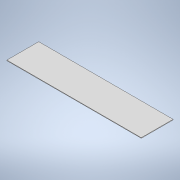
# Autodesk Inventor part: placa grande
Saved by Autodesk Inventor 2021.2 (Build 252289000, 289)
## iProperties
Created: 2021-04-23
Part Number: placa grande
Material: Genérico
Document SubType Name: Modeling
Designer: equip
Density: 1 g/cm^3
Appearance: Valor por defecto
Author: equip
Autodesk Inventor part; units mm, degrees
ref_plane "YZ Plane" through (0, 0, 0) normal (1, 0, 0) x (0, 1, 0)
ref_plane "XZ Plane" through (0, 0, 0) normal (0, 1, 0) x (-1, 0, 0)
ref_plane "XY Plane" through (0, 0, 0) normal (0, 0, 1) x (1, 0, 0)
sketch "Boceto1" plane through (0, 0, 0) normal (0, 1, 0) x (-1, 0, 0)
  line L0 (0, 0) -> (2365, 0)
  line L1 (2365, 0) -> (2365, 560)
  line L2 (2365, 560) -> (0, 560)
  line L3 (0, 560) -> (0, 0)
  dimension "d0" = 2365
  dimension "d1" = 560
  constraints: 8 end point, 2 parallel, 1 horizontal, 1 perpendicular
  measures "d0" distance of L2.end L1.end
  measures "d1" distance of L1.end L0.end
extrude "Extrusión1" add sketch "Boceto1" along normal blind 10
